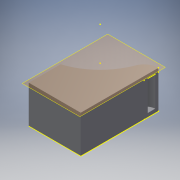
# Autodesk Inventor part: guide
Saved by Autodesk Inventor 2016 (Build 200138000, 138)
## iProperties
Created: 2016-01-18
Part Number: guide
Material: Generic
Document SubType Name: Modeling
Designer: Erwin Ried
Density: 1 g/cm^3
Appearance: Default
Author: Erwin Ried
Autodesk Inventor part; units mm, degrees
ref_plane "YZ Plane" through (0, 0, 0) normal (1, 0, 0) x (0, 1, 0)
ref_plane "XZ Plane" through (0, 0, 0) normal (0, 1, 0) x (-1, 0, 0)
ref_plane "XY Plane" through (0, 0, 0) normal (0, 0, 1) x (1, 0, 0)
ref_plane "Work Plane1" through (0, 0, 0) normal (0, 0, 1) x (1, 0, 0)
sketch "Sketch1" plane through (0, 0, 0) normal (0, 0, 1) x (1, 0, 0)
  line L0 (-27.74, -41.4747) -> (0, -41.4747)
  arc A0 (-27.74, -24.4747) -> (-7.389, -5.4576) centre (-37.6712, 6.5509) ccw
  arc A1 (0, 0) -> (-7.389, -5.4576) centre (-0.0343, -7.6843) ccw
  line L1 (0, 0) -> (0, -41.4747)
  line L2 (-27.74, -24.4747) -> (-27.74, -41.4747)
  constraints: 6 end point, 4 point on circle, 2 centre point, 1 horizontal, 1 parallel, 1 perpendicular, 3 other
extrude "Extrusion1" add sketch "Sketch1" against normal blind 20
sketch "Sketch2" plane through (0, 0, 0) normal (1, 0, 0) x (0, 0, -1)
  point P0 (0, 0)
shell "Shell1" thickness 2 removed faces 1 at (-27.74, -30.1414, -6.6667)
sketch "Sketch3" plane through (0, 0, 0) normal (1, 0, 0) x (0, 0, -1)
  line L0 (1.5487, -2.9607) -> (1.5603, -2.908) projected
  line L1 (1.5603, -2.908) -> (1.6355, -2.6468) projected
  line L2 (1.6355, -2.6468) -> (1.7427, -2.3861) projected
  line L3 (1.7427, -2.3861) -> (1.7557, -2.3596) projected
  line L4 (1.7557, -2.3596) -> (1.8896, -2.12) projected
  line L5 (1.8896, -2.12) -> (1.9914, -1.9634) projected
  line L6 (1.9914, -1.9634) -> (2.0599, -1.8668) projected
  line L7 (2.0599, -1.8668) -> (2.2163, -1.6705) projected
  line L8 (2.2163, -1.6705) -> (2.2384, -1.6452) projected
  line L9 (2.2384, -1.6452) -> (2.4301, -1.4489) projected
  line L10 (2.4301, -1.4489) -> (2.5857, -1.304) projected
  line L11 (2.5857, -1.304) -> (2.6284, -1.2661) projected
  line L12 (2.6284, -1.2661) -> (2.7517, -1.1606) projected
  line L13 (2.7517, -1.1606) -> (2.8143, -1.1094) projected
  line L14 (2.8143, -1.1094) -> (2.9296, -1.0186) projected
  line L15 (2.9296, -1.0186) -> (2.9933, -0.9699) projected
  line L16 (2.9933, -0.9699) -> (3.1154, -0.8782) projected
  line L17 (3.1154, -0.8782) -> (3.166, -0.8406) projected
  line L18 (3.166, -0.8406) -> (3.3051, -0.7395) projected
  line L19 (3.3051, -0.7395) -> (3.3348, -0.7182) projected
  line L20 (3.3348, -0.7182) -> (3.5, -0.6024) projected
  line L21 (3.5, -0.6024) -> (16.5, -0.6024) projected
  line L22 (16.5, -0.6024) -> (16.6509, -0.7063) projected
  line L23 (16.6509, -0.7063) -> (16.798, -0.8118) projected
  line L24 (16.798, -0.8118) -> (16.8324, -0.8371) projected
  line L25 (16.8324, -0.8371) -> (16.9413, -0.9188) projected
  line L26 (16.9413, -0.9188) -> (17.0058, -0.9683) projected
  line L27 (17.0058, -0.9683) -> (17.0809, -1.0271) projected
  line L28 (17.0809, -1.0271) -> (17.185, -1.1098) projected
  line L29 (17.185, -1.1098) -> (17.2176, -1.1363) projected
  line L30 (17.2176, -1.1363) -> (17.3504, -1.247) projected
  line L31 (17.3504, -1.247) -> (17.372, -1.2657) projected
  line L32 (17.372, -1.2657) -> (17.4776, -1.3607) projected
  line L33 (17.4776, -1.3607) -> (17.569, -1.4485) projected
  line L34 (17.569, -1.4485) -> (17.5985, -1.4777) projected
  line L35 (17.5985, -1.4777) -> (17.7841, -1.6747) projected
  line L36 (17.7841, -1.6747) -> (17.8234, -1.7202) projected
  line L37 (17.8234, -1.7202) -> (17.9262, -1.8486) projected
  line L38 (17.9262, -1.8486) -> (18.0068, -1.9599) projected
  line L39 (18.0068, -1.9599) -> (18.0235, -1.9841) projected
  line L40 (18.0235, -1.9841) -> (18.1149, -2.1252) projected
  line L41 (18.1149, -2.1252) -> (18.1977, -2.2689) projected
  line L42 (18.1977, -2.2689) -> (18.2436, -2.3579) projected
  line L43 (18.2436, -2.3579) -> (18.2696, -2.4125) projected
  line L44 (18.2696, -2.4125) -> (18.3312, -2.5574) projected
  line L45 (18.3312, -2.5574) -> (18.4255, -2.8495) projected
  line L46 (18.4255, -2.8495) -> (18.4521, -2.9635) projected
  line L47 (18.4521, -2.9635) -> (18.4818, -3.1403) projected
  line L48 (18.4818, -3.1403) -> (18.5, -3.4308) projected
  line L49 (18.5, -5.7085) -> (18.5, -3.4308) projected
  line L50 (18.5, -5.7085) -> (20, -5.7085) projected
  line L51 (20, -5.7085) -> (20, 0) projected
  line L52 (0, 0) -> (20, 0) projected
  line L53 (0, -5.7085) -> (0, 0) projected
  line L54 (0, -5.7085) -> (1.5, -5.7085) projected
  line L55 (1.5, -5.7085) -> (1.5, -3.4308) projected
  line L56 (1.5, -3.4308) -> (1.5149, -3.1693) projected
  line L57 (1.5149, -3.1693) -> (1.5487, -2.9607) projected
  line L58 (0, -5.7085) -> (20, -5.7085)
  line L59 (0, -5.4576) -> (20, -5.4576) projected
  line L60 (2, -9.7085) -> (18, -9.7085)
  line L61 (18, -9.7085) -> (18, -1.7085)
  line L62 (18, -1.7085) -> (2, -1.7085)
  line L63 (2, -1.7085) -> (2, -9.7085)
  line L64 (2, -9.7085) -> (18, -1.7085) construction
  line L65 (18, -9.7085) -> (2, -1.7085) construction
  line L66 (18, -6.1101) -> (18, -2.3506) projected
  line L67 (2, -1.7085) -> (18, -1.7085)
  line L68 (18, -1.7085) -> (18, -5.7085)
  line L69 (18, -5.7085) -> (2, -5.7085)
  line L70 (2, -5.7085) -> (2, -1.7085)
  point P0 (10, -5.7085)
  dimension "d6" = 8
  constraints: 22 end point, 5 parallel, 3 midpoint, 2 perpendicular, 2 point on line, 1 horizontal
  measures "d6" distance of L61.end L60.end
extrude "Extrusion2" cut sketch "Sketch3" against normal blind 2 contours L63 L6 L7 L62 L36 L37 L38 L61 L59 | L59 L61 L58 L63 | L63 L62 L7 L6 | L38 L37 L36 L62 L61
sketch "Sketch4" plane through (-14.2142, -39.4747, -2) normal (0, 0, -1) x (-1, 0, 0)
  point P0 (-14.2142, 39.4747)
sketch "Sketch5" plane through (-14.2142, -39.4747, -2) normal (0, 0, -1) x (-1, 0, 0)
  line L0 (13.5258, 0) -> (-12.2142, 0) projected
  line L1 (13.5258, 12.9062) -> (13.5258, 0) projected
  arc A0 (-8.7179, 33.3646) -> (13.5258, 12.9062) centre (23.4569, 46.0256) ccw projected
  arc A1 (-8.7179, 33.3646) -> (-12.2142, 37.1241) centre (-14.1799, 31.7904) ccw projected
  line L2 (-12.2142, 37.1241) -> (-12.2142, 37.7662) projected
  line L3 (-14.2142, 37.7662) -> (-12.2142, 37.7662) projected
  line L4 (-14.2142, 33.7662) -> (-14.2142, 37.7662) projected
  line L5 (-14.2142, 33.7662) -> (-12.2142, 33.7662) projected
  line L6 (-12.2142, 0) -> (-12.2142, 33.7662) projected
  point P0 (-14.2142, 39.4747)
fillet "Fillet1" radius 3 1 edges at (-2, -2.3506, -10)
fillet "Fillet2" radius 5.5 2 edges at (-2, -1.7085, -10) (-2, -1.7085, -2)
fillet "Fillet5" [suppressed]
sketch "Sketch6" plane through (-27.74, -39.4747, -18) normal (0, 0, 1) x (1, 0, 0)
  line L0 (0, 0) -> (25.74, 0) projected
  line L1 (0, 0) -> (0, 12.9062) projected
  line L2 (0, 1) -> (-44, 1) projected
  arc A0 (11.0973, 0) -> (14.6461, 2.1546) centre (11.0973, 4) ccw projected
  line L3 (0, 1) -> (11.0973, 0)
  line L4 (11.0973, 0) -> (0, 0)
  point P0 (27.74, 39.4747)
  point P1 (0, 10.8234)
  constraints: 4 end point, 1 parallel, 1 tangent
extrude "Extrusion3" add sketch "Sketch6" along normal blind 16
sketch "Sketch8" plane through (0, 0, -20) normal (0, 0, -1) x (-1, 0, 0)
  line L0 (0, -41.4747) -> (27.74, -41.4747) projected
  line L1 (27.74, -41.4747) -> (27.74, -24.4747) projected
  arc A0 (7.389, -5.4576) -> (27.74, -24.4747) centre (37.6712, 6.5509) ccw projected
  arc A1 (7.389, -5.4576) -> (0, 0) centre (0.0343, -7.6843) ccw projected
  line L2 (0, 0) -> (0, -41.4747) projected
body "Solid1"
